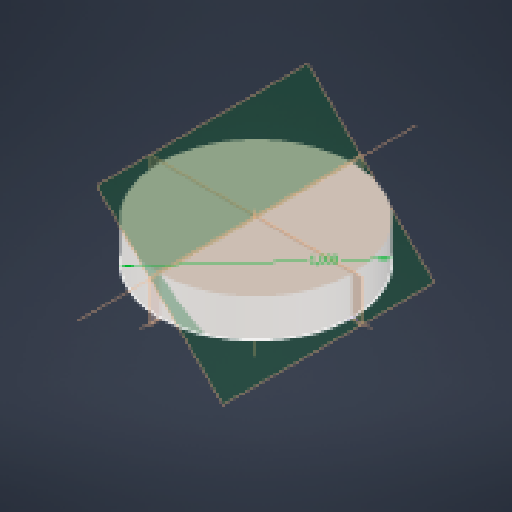
# Autodesk Inventor part: 1in_5mm_mir
Saved by Autodesk Inventor 2026.1 (Build 301233000, 233)
## iProperties
Created: 2019-05-24
Part Number: 1in_5mm_mir
Material: Generisch
Document SubType Name: Modeling
Designer: Julian
Density: 1 g/cm^3
Appearance: Vorgabe
Mass: 2.57407 g
Surface Area: 14.1878 cm^2
Volume: 2.57407 cm^3
Author: Julian
Autodesk Inventor part; units mm, degrees
ref_plane "YZ Plane" through (0, 0, 0) normal (1, 0, 0) x (0, 1, 0)
ref_plane "XZ Plane" through (0, 0, 0) normal (0, 1, 0) x (-1, 0, 0)
sketch "Sketch1" plane through (0, 0, 0) normal (0, 1, 0) x (-1, 0, 0)
  circle A0 centre (0, 0) radius 12.7
  point P0 (-12.7, 0)
  point P1 (0, -12.7)
  dimension "d0" = 25.4
  constraints: 2 coincident, 2 point on circle, 1 centre point
  measures "d0" diameter of A0
extrude "Extrusion1" add sketch "Sketch1" along normal blind 5.08
ref_plane "Work Plane11" through (0, 0, 0) normal (-1, 0, 0) x (0, -1, 0)
ref_plane "Work Plane12" through (0, 0, 0) normal (0, 0, 1) x (0, -1, 0)
ref_plane "Work Plane13" through (0, 5.08, 0) normal (-0.7071, 0.7071, 0) x (0, 0, 1)
ref_plane "Work Plane14" through (0, 5.08, 0) normal (-0.7071, -0.7071, 0) x (0, 0, 1)
ref_plane "Work Plane15" through (0, 0, 0) normal (0, 0, 1) x (0, -1, 0)
ref_plane "Work Plane16" through (0, 0, -12.7) normal (1, 0, 0) x (0, 0, 1)
body "Solid1"
